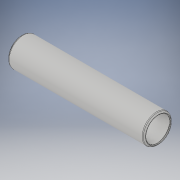
# Autodesk Inventor part: 02R-2.8870
Saved by Autodesk Inventor 2019 (Build 230136000, 136)
## iProperties
Created: 2023-02-02
Part Number: 02R-2.8870
Material: Generic
Catalog Web Link: www.cadenas.de
Description: Tube-Original Line - Standard Air Cylinders
Vendor: BIMBA
Document SubType Name: Modeling
Designer: psAdmin
Manufacturer: BIMBA
Mass: 1.91629 g
Surface Area: 71.1165 cm^2
Volume: 1.91629 cm^3
Density: 1 g/cm^3
Appearance: PSOLRGB-180-180-180
Category: PARTsolutions
Company: BIMBA
Title: 02R-2.8870
Author: Cadenas PARTsolutions
Comments: Original Line - Standard Air Cylinders
PSOL_IDENT_0: {$CADENAS_DATA/23d-libs/bimba/bimba_brand/bimba_imperial/bimba_full_line/original_line_cylinders/sta
PSOL_IDENT_1: ndard_air_cylinders/tube.prj},199 {VTYP=3D},{NB=02R-2.8870},{LINA=02R-2.8870},{NN=Tube},{DATE=26.01.
PSOL_IDENT_2: 2023 11:43:57},{GEOMDATE=25.01.2023 10:00:00},{VERSION=},{LINEID=30},{WBVAR=MNT,ACTING,NR,L,FOURHOLE
PSOL_IDENT_3: S,SR,K},{WBNUMERIC=L,FOURHOLES}  {NB=02R-2.8870},{LINA=02R-2.8870},{KT=DUMMY},{PN=02R-2.8870},{BORE=
PSOL_IDENT_4: 0.56250000},{BOREPN=02},{MNT=},{MNTALG='' , 'Front Nose'},{ACTING=R},{ACTINGALG= '' , 'Single Acting'
PSOL_IDENT_5: , 'R' , 'Reverse/Double Acting' },{NR=},{NRALG= '' , 'N/A' },{L=2.8870},{OD=0.6150},{ODN=0.6150},{O
PSOL_IDENT_6: DP=0.6150},{ODB=0.0000},{ID=0.5725},{DV=0.00000000},{LV=0.00000000},{LV1=0.00000000},{G=0.0250},{FOU
PSOL_IDENT_7: RHOLES=0},{AA=0.3750},{BB=0.0940},{SR=},{SRALG= 'C' , 'Carbon Steel Rod' , 'SR' , '303 Stainless Ste
PSOL_IDENT_8: el Rod' , '' , '303 Stainless Steel Rod'},{KALG= '', 'Standard' , 'K' , 'Ports Rotated 90deg' },{K=}
NB: 02R-2.8870
NN: Tube
NT: Original Line - Standard Air Cylinders
NBSYN: $PN.
LINA: 02R-2.8870
CATALOG: Bimba Products
BORE: 0
BOREPN: 02
MNT: Front Nose
MNTALG: '' , 'Front Nose'
ACTING: Reverse/Double Acting
NR: N/A
L: 2.887
ODN: 0.615
ODP: 0.615
ODB: 0
ID: 0.5725
DV: 0
LV: 0
LV1: 0
G: 0.025
FOURHOLES: 0
AA: 0.375
BB: 0.094
SR: 303 Stainless Steel Rod
K: Standard
SUPPLIER: BIMBA
ARTICLENO: 02R-2.8870
BOMINFO: 02R-2.8870
CREATOR: CADENAS GmbH
Autodesk Inventor part; units mm, degrees
sketch "Sketch_1" plane through (0, 0, 0) normal (0, 0, 1) x (1, 0, 0)
  line L0 (73.3298, 0) -> (0, 0)
  arc A0 (-0.518, 7.0158) -> (-0.518, 6.8362) centre (-0.4282, 6.926) ccw
  line L1 (-0.518, 6.8362) -> (-0.3175, 6.6357)
  line L2 (-0.3175, 6.6357) -> (0, 6.6357)
  line L3 (0, 6.6357) -> (0.635, 7.2708)
  line L4 (0.635, 7.2708) -> (72.6948, 7.2708)
  line L5 (72.6948, 7.2708) -> (73.3298, 6.6357)
  line L6 (73.3298, 6.6357) -> (73.6473, 6.6357)
  line L7 (73.6473, 6.6357) -> (73.8478, 6.8362)
  arc A1 (73.8478, 6.8362) -> (73.8478, 7.0158) centre (73.758, 6.926) ccw
  line L8 (73.8478, 7.0158) -> (73.2391, 7.6245)
  arc A2 (73.2391, 7.6245) -> (72.79, 7.8105) centre (72.79, 7.1755) ccw
  line L9 (72.79, 7.8105) -> (0.5398, 7.8105)
  arc A3 (0.5398, 7.8105) -> (0.0907, 7.6245) centre (0.5398, 7.1755) ccw
  line L10 (0.0907, 7.6245) -> (-0.518, 7.0158)
  constraints: 22 end point, 8 point on circle, 4 centre point
revolve "Revolution1" add sketch "Sketch_1" angle 360 about axis through (73.3298, 0, 0) along (1, 0, 0)
ref_plane "cp1_XY" through (36.6649, 0, 7.8105) normal (1, 0, 0) x (0, 0, -1)
ref_plane "cp1_YZ" through (36.6649, 0, 7.8105) normal (0, 0, -1) x (0, 1, 0)
ref_plane "cp1_ZX" through (36.6649, 0, 7.8105) normal (0, 1, 0) x (1, 0, 0)
ref_plane "cp2_XY" through (36.6649, -7.8105, 0) normal (1, 0, 0) x (0, 0, -1)
ref_plane "cp2_YZ" through (36.6649, -7.8105, 0) normal (0, 0, -1) x (0, 1, 0)
ref_plane "cp2_ZX" through (36.6649, -7.8105, 0) normal (0, 1, 0) x (1, 0, 0)
ref_plane "cp3_XY" through (36.6649, 0, -7.8105) normal (1, 0, 0) x (0, 0, -1)
ref_plane "cp3_YZ" through (36.6649, 0, -7.8105) normal (0, 0, -1) x (0, 1, 0)
ref_plane "cp3_ZX" through (36.6649, 0, -7.8105) normal (0, 1, 0) x (1, 0, 0)
ref_plane "cp4_XY" through (36.6649, 7.8105, 0) normal (1, 0, 0) x (0, 0, -1)
ref_plane "cp4_YZ" through (36.6649, 7.8105, 0) normal (0, 0, -1) x (0, 1, 0)
ref_plane "cp4_ZX" through (36.6649, 7.8105, 0) normal (0, 1, 0) x (1, 0, 0)
ref_plane "tube_front_XY" through (0, 0, 0) normal (1, 0, 0) x (0, 0, -1)
ref_plane "tube_front_YZ" through (0, 0, 0) normal (0, 0, -1) x (0, 1, 0)
ref_plane "tube_front_ZX" through (0, 0, 0) normal (0, 1, 0) x (1, 0, 0)
ref_plane "tube_rear_XY" through (73.3298, 0, 0) normal (1, 0, 0) x (0, 0, -1)
ref_plane "tube_rear_YZ" through (73.3298, 0, 0) normal (0, 0, -1) x (0, 1, 0)
ref_plane "tube_rear_ZX" through (73.3298, 0, 0) normal (0, 1, 0) x (1, 0, 0)
body "Solid1"
